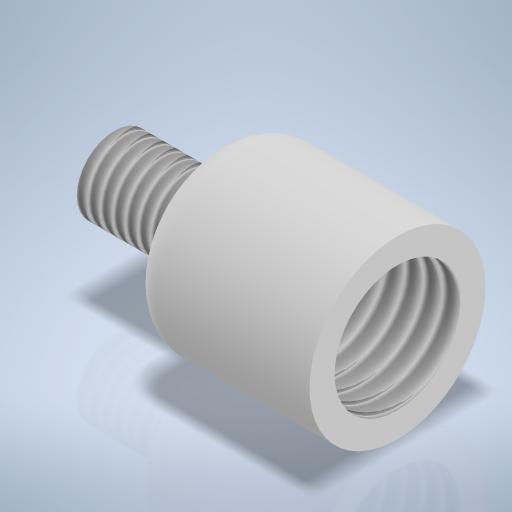
# Autodesk Inventor part: 1071
Saved by Autodesk Inventor 2024 (Build 280153000, 153)
## iProperties
Created: 2024-06-07
Part Number: 1071
Material: Generisch
Document SubType Name: Modeling
Designer: ffogue
Density: 1 g/cm^3
Appearance: Vorgabe
Author: ffogue
Autodesk Inventor part; units mm, degrees
ref_plane "YZ Plane" through (0, 0, 0) normal (1, 0, 0) x (0, 1, 0)
ref_plane "XZ Plane" through (0, 0, 0) normal (0, 1, 0) x (-1, 0, 0)
ref_plane "XY Plane" through (0, 0, 0) normal (0, 0, 1) x (1, 0, 0)
sketch "Skizze1" plane through (0, 0, 0) normal (0, 1, 0) x (-1, 0, 0)
  line L0 (0, 0) -> (0, 3)
  line L1 (0, 3) -> (-8, 3)
  line L2 (-8, 3) -> (-8, 4.5)
  line L3 (-10.5, 7) -> (-22.5, 7)
  line L4 (-22.5, 7) -> (-22.5, 0)
  line L5 (-22.5, 0) -> (0, 0)
  arc A0 (-8, 4.5) -> (-10.5, 7) centre (-10.5, 4.5) ccw
  point P0 (-8, 7)
  dimension "d0" = 6
  dimension "d1" = 8
  dimension "d2" = 14.5
  dimension "d3" = 14
  dimension "d4" = 2.5
  constraints: 12 end point, 5 perpendicular, 2 point on circle, 2 point on line, 2 tangent, 1 centre point, 1 vertical
  measures "d0" diameter of L1 L5
  measures "d1" distance of L0.end L1.end
  measures "d2" distance of point (-8, 7) L3.end
  measures "d3" diameter of L3 L5
  measures "d4" radius of A0
revolve "Umdrehung1" add sketch "Skizze1" angle 360 about axis through (22.5, 0, 0) along (-1, 0, 0)
thread "Gewinde1" size "M6x1" class "6g" standard "ISO Metric profile" length 8
sketch "Skizze2" plane through (0, 0, 0) normal (0, 1, 0) x (-1, 0, 0)
  line L0 (0, 0) -> (-22.5, 0)
  line L1 (-22.5, -7) -> (-22.5, 7) projected
  line L2 (0, -1.5) -> (-9.5, -1.5)
  line L3 (0, -1.5) -> (0, 0)
  line L4 (0, -3) -> (0, 3) projected
  line L5 (-11, -5) -> (-22.5, -5)
  line L6 (-9.5, -1.5) -> (-11, -5)
  line L7 (-22.5, -5) -> (-22.5, 0)
  dimension "d8" = 3
  dimension "d9" = 9.5
  dimension "d12" = 10
  dimension "d13" = 11.5
  constraints: 12 end point, 1 collinear, 1 horizontal, 1 midpoint, 1 perpendicular, 1 point on line, 1 vertical
  measures "d8" diameter of L2 L0
  measures "d9" distance of L2.start L2.end
  measures "d12" diameter of L5 L0
  measures "d13" distance of L5.start L5.end
revolve "Umdrehung2" cut sketch "Skizze2" angle 360 about axis through (0, 0, 0) along (1, 0, 0)
fillet "Rundung1" radius 2 1 edges at (11, 0, 5)
thread "Gewinde2" size "M10x1.5" class "6H" standard "ISO Metric profile" length 10.181
